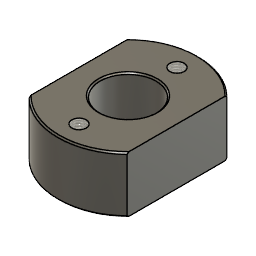
P1 (Autodesk Fusion 360 design; units mm, degrees)
part number: 2026-08-20-08-42-54-312
Autodesk Fusion 360 part; units mm, degrees
sketch "Sketch1" plane through (0, 0, 0) normal (0, 1, 0) x (1, 0, 0)
  circle A0 centre (0, 0) radius 20
  line L0 (-35, 35.7071) -> (-35, -35.7071)
  line L1 (0, 0) -> (0, 70.7339) construction
  line L2 (35, 35.7071) -> (35, -35.7071)
  arc A1 (-35, -35.7071) -> (35, -35.7071) centre (0, 0) ccw
  arc A2 (35, 35.7071) -> (-35, 35.7071) centre (0, 0) ccw
  dimension "d1" = 40
  dimension "d2" = 100
  dimension "d3" = 70
  dimension "d6" = 35
  constraint coincident A0.centre L1.start
  constraint vertical L0
  constraint vertical L1
  constraint concentric A1 A2
  measures "d1" diameter of A0
  measures "d2" diameter of A1
  measures "d3" distance of L0 L2
  measures "d6" distance of A0.centre L2
extrude "Extrude1" add sketch "Sketch1" along normal mid plane 40
sketch "Sketch2" plane through (0, 20, 0) normal (0, 1, 0) x (-1, 0, 0)
  circle A0 centre (0, 0) radius 20
  arc A1 (-35, -35.7071) -> (35, -35.7071) centre (0, 0) ccw
  line L0 (35, -35.7071) -> (35, 35.7071)
  arc A2 (35, 35.7071) -> (-35, 35.7071) centre (0, 0) ccw
  line L1 (-35, 35.7071) -> (-35, -35.7071)
  circle A3 centre (0, -35) radius 5
  line L2 (0, 0) -> (45, 0) construction
  circle A4 centre (0, 35) radius 5
  dimension "d7" = 10
  dimension "d8" = 35
  constraint coincident A0.centre A1.centre
  constraint perpendicular L0 L2
  constraint symmetric A3 L2 A4
  measures "d7" diameter of A3
  measures "d8" distance of A3.centre L2
extrude "Extrude2" cut sketch "Sketch2" against normal blind 80 contours A3 | A4
chamfer "Chamfer1" distance 1 angle 45 3 edges at (0, 20, -50) (0, 20, 50) (-18.6465, 20, -7.2323)
chamfer "Chamfer1" distance 1 angle 45 3 edges at (0, -20, -50) (0, -20, 50) (-18.6465, -20, 7.2323)
hole "Hole1" at (0, -20, -35) direction (0, 1, 0) diameter 10.274 end through all
thread "Thread1" "ISO Metric profile 12.0 M12x1.75 M12x1.75 6H" thread offset 0 thread depth 7.4
hole "Hole2" at (0, -20, 35) direction (0, 1, 0) diameter 10.274 end through all
thread "Thread2" "ISO Metric profile 12.0 M12x1.75 M12x1.75 6H" thread offset 0 thread depth 7.4
chamfer "Chamfer2" distance 2 angle 45 2 edges at (1.8575, -20, -30.2109) (1.8575, -20, 39.7891)
